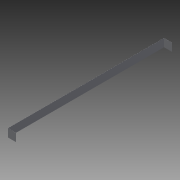
# Autodesk Inventor part: Cloth
Saved by Autodesk Inventor 2013 (Build 170138000, 138)
## iProperties
Created: 2014-01-21
Part Number: Cloth
Material: Generic
Document SubType Name: Modeling
Designer: RobertB
Density: 1 g/cm^3
Author: RobertB
Autodesk Inventor part; units mm, degrees
ref_plane "YZ Plane" through (0, 0, 0) normal (1, 0, 0) x (0, 1, 0)
ref_plane "XZ Plane" through (0, 0, 0) normal (0, 1, 0) x (-1, 0, 0)
ref_plane "XY Plane" through (0, 0, 0) normal (0, 0, 1) x (1, 0, 0)
sketch "Sketch1" plane through (0, 0, 0) normal (1, 0, 0) x (0, 1, 0)
  line L0 (-12.7, 247.65) -> (12.7, 247.65)
  line L1 (12.7, 247.65) -> (12.7, -247.65)
  line L2 (12.7, -247.65) -> (-12.7, -247.65)
  line L3 (-12.7, -247.65) -> (-12.7, 247.65)
  line L4 (-12.7, 247.65) -> (12.7, -247.65) construction
  line L5 (12.7, 247.65) -> (-12.7, -247.65) construction
  point P0 (0, 0)
  dimension "d0" = 25.4
  dimension "d1" = 495.3
  constraints: 12 end point, 2 midpoint, 2 parallel, 1 horizontal, 1 perpendicular
  measures "d0" distance of L1.end L2.end
  measures "d1" distance of L0.end L1.end
extrude "Extrusion1" add sketch "Sketch1" along normal blind 0.254
sketch "Sketch2" plane through (0.254, 0, 0) normal (1, 0, 0) x (0, 0, -1)
  line L0 (-247.65, 12.7) -> (-247.904, 12.7)
  line L1 (-247.904, 12.7) -> (-247.904, -12.7)
  line L2 (-247.904, -12.7) -> (-247.65, -12.7)
  line L3 (-247.65, -12.7) -> (-247.65, 12.7)
  line L4 (247.65, 12.7) -> (247.904, 12.7)
  line L5 (247.904, 12.7) -> (247.904, -12.7)
  line L6 (247.904, -12.7) -> (247.65, -12.7)
  line L7 (247.65, -12.7) -> (247.65, 12.7)
  point P0 (0, 0)
  dimension "d4" = 0.254
  dimension "d5" = 25.4
  dimension "d6" = 0.254
  dimension "d7" = 25.4
  constraints: 16 end point, 4 parallel, 2 horizontal, 2 perpendicular
  measures "d4" distance of L2.end L1.end
  measures "d5" distance of L1.end L0.end
  measures "d6" distance of L5.end L6.end
  measures "d7" distance of L4.end L5.end
extrude "Extrusion2" add sketch "Sketch2" along normal blind 25.4
body "Solid1"
